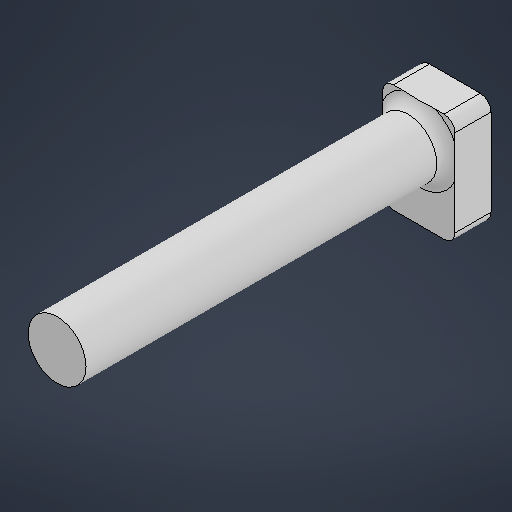
# Autodesk Inventor part: slidev
Saved by Autodesk Inventor 2026 (Build 300175050, 175E)
## iProperties
Created: 2025-09-02
Part Number: slidev
Material: 一般
Document SubType Name: Modeling
Designer: ka0n7
Density: 1 g/cm^3
Appearance: 既定
Author: ka0n7
Autodesk Inventor part; units mm, degrees
ref_plane "YZ Plane" through (0, 0, 0) normal (1, 0, 0) x (0, 1, 0)
ref_plane "XZ Plane" through (0, 0, 0) normal (0, 1, 0) x (-1, 0, 0)
ref_plane "XY Plane" through (0, 0, 0) normal (0, 0, 1) x (1, 0, 0)
sketch "スケッチ1" plane through (0, 0, 0) normal (0, 0, 1) x (1, 0, 0)
  line L0 (5, 7.5) -> (-5, 7.5)
  line L1 (-5, 7.5) -> (-5, -7.5)
  line L2 (-5, -7.5) -> (5, -7.5)
  line L3 (5, -7.5) -> (5, 7.5)
  line L4 (5, 7.5) -> (-5, -7.5) construction
  line L5 (-5, 7.5) -> (5, -7.5) construction
  point P0 (0, 0)
  dimension "d0" = 10
  dimension "d1" = 15
  constraints: 12 end point, 2 midpoint, 2 parallel, 1 horizontal, 1 perpendicular
  measures "d0" distance of L2.end L1.end
  measures "d1" distance of L2.end L0.start
extrude "押し出し1" add sketch "スケッチ1" along normal blind 5
sketch "スケッチ2" plane through (0, 0, 5) normal (0, 0, 1) x (1, 0, 0)
  line L0 (0, 0) -> (0, 2.5)
  circle A0 centre (0, 2.5) radius 4
  dimension "d4" = 2.5
  dimension "d5" = 8
  constraints: 2 end point, 1 centre point, 1 coincident, 1 vertical
  measures "d4" distance of L0.start L0.end
  measures "d5" diameter of A0
extrude "押し出し2" add sketch "スケッチ2" along normal blind 50
fillet "フィレット1" radius 1.5 1 edges at (-4, 2.5, 5)
fillet "フィレット2" radius 1.5 4 edges at (5, 7.5, 2.5) (-5, 7.5, 2.5) (5, -7.5, 2.5) (-5, -7.5, 2.5)
